Autodesk Inventor part; units mm, degrees
(part 2 of 2)
  circle A1101 centre (-5.5, 0.5) radius 0.125
  circle A1102 centre (-5.5, 1) radius 0.125
  circle A1103 centre (-5.5, 1.5) radius 0.125
  circle A1104 centre (-5.5, 2) radius 0.125
  circle A1105 centre (-5.5, 2.5) radius 0.125
  circle A1106 centre (-5.5, 3) radius 0.125
  circle A1107 centre (-5.5, 5) radius 0.125
  circle A1108 centre (-5.5, 5.5) radius 0.125
  circle A1109 centre (-5.5, 6) radius 0.125
  circle A1110 centre (-5.5, 6.5) radius 0.125
  line L13 (-6, -9) -> (-6, 0) construction
  circle A1111 centre (-6, -5.5) radius 0.125
  circle A1112 centre (-6, -5) radius 0.125
  circle A1113 centre (-6, -3.5) radius 0.125
  circle A1114 centre (-6, -4) radius 0.125
  circle A1115 centre (-6, -4.5) radius 0.125
  circle A1116 centre (-6, -7.5) radius 0.125
  circle A1117 centre (-6, -7) radius 0.125
  circle A1118 centre (-6, -6.5) radius 0.125
  circle A1119 centre (-6, -6) radius 0.125
  circle A1120 centre (-6, -3) radius 0.125
  circle A1121 centre (-6, -2.5) radius 0.125
  circle A1122 centre (-6, -2) radius 0.125
  circle A1123 centre (-6, -1.5) radius 0.125
  circle A1124 centre (-6, 0) radius 0.125
  circle A1125 centre (-6, -0.5) radius 0.125
  circle A1126 centre (-6, -1) radius 0.125
  circle A1127 centre (-6, -9) radius 0.125
  circle A1128 centre (-6, -8.5) radius 0.125
  circle A1129 centre (-6, -8) radius 0.125
  circle A1130 centre (-6, 3.5) radius 0.125
  circle A1131 centre (-6, 4) radius 0.125
  circle A1132 centre (-6, 4.5) radius 0.125
  circle A1133 centre (-6, 7) radius 0.125
  circle A1134 centre (-6, 7.5) radius 0.125
  circle A1135 centre (-6, 8) radius 0.125
  circle A1136 centre (-6, 8.5) radius 0.125
  circle A1137 centre (-6, 9) radius 0.125
  circle A1138 centre (-6, 0.5) radius 0.125
  circle A1139 centre (-6, 1) radius 0.125
  circle A1140 centre (-6, 1.5) radius 0.125
  circle A1141 centre (-6, 2) radius 0.125
  circle A1142 centre (-6, 2.5) radius 0.125
  circle A1143 centre (-6, 3) radius 0.125
  circle A1144 centre (-6, 5) radius 0.125
  circle A1145 centre (-6, 5.5) radius 0.125
  circle A1146 centre (-6, 6) radius 0.125
  circle A1147 centre (-6, 6.5) radius 0.125
  line L14 (-6.5, -9) -> (-6.5, 0) construction
  circle A1148 centre (-6.5, -5.5) radius 0.125
  circle A1149 centre (-6.5, -5) radius 0.125
  circle A1150 centre (-6.5, -3.5) radius 0.125
  circle A1151 centre (-6.5, -4) radius 0.125
  circle A1152 centre (-6.5, -4.5) radius 0.125
  circle A1153 centre (-6.5, -7.5) radius 0.125
  circle A1154 centre (-6.5, -7) radius 0.125
  circle A1155 centre (-6.5, -6.5) radius 0.125
  circle A1156 centre (-6.5, -6) radius 0.125
  circle A1157 centre (-6.5, -3) radius 0.125
  circle A1158 centre (-6.5, -2.5) radius 0.125
  circle A1159 centre (-6.5, -2) radius 0.125
  circle A1160 centre (-6.5, -1.5) radius 0.125
  circle A1161 centre (-6.5, 0) radius 0.125
  circle A1162 centre (-6.5, -0.5) radius 0.125
  circle A1163 centre (-6.5, -1) radius 0.125
  circle A1164 centre (-6.5, -9) radius 0.125
  circle A1165 centre (-6.5, -8.5) radius 0.125
  circle A1166 centre (-6.5, -8) radius 0.125
  circle A1167 centre (-6.5, 3.5) radius 0.125
  circle A1168 centre (-6.5, 4) radius 0.125
  circle A1169 centre (-6.5, 4.5) radius 0.125
  circle A1170 centre (-6.5, 7) radius 0.125
  circle A1171 centre (-6.5, 7.5) radius 0.125
  circle A1172 centre (-6.5, 8) radius 0.125
  circle A1173 centre (-6.5, 8.5) radius 0.125
  circle A1174 centre (-6.5, 9) radius 0.125
  circle A1175 centre (-6.5, 0.5) radius 0.125
  circle A1176 centre (-6.5, 1) radius 0.125
  circle A1177 centre (-6.5, 1.5) radius 0.125
  circle A1178 centre (-6.5, 2) radius 0.125
  circle A1179 centre (-6.5, 2.5) radius 0.125
  circle A1180 centre (-6.5, 3) radius 0.125
  circle A1181 centre (-6.5, 5) radius 0.125
  circle A1182 centre (-6.5, 5.5) radius 0.125
  circle A1183 centre (-6.5, 6) radius 0.125
  circle A1184 centre (-6.5, 6.5) radius 0.125
  line L15 (-7, -9) -> (-7, 0) construction
  circle A1185 centre (-7, -5.5) radius 0.125
  circle A1186 centre (-7, -5) radius 0.125
  circle A1187 centre (-7, -3.5) radius 0.125
  circle A1188 centre (-7, -4) radius 0.125
  circle A1189 centre (-7, -4.5) radius 0.125
  circle A1190 centre (-7, -7.5) radius 0.125
  circle A1191 centre (-7, -7) radius 0.125
  circle A1192 centre (-7, -6.5) radius 0.125
  circle A1193 centre (-7, -6) radius 0.125
  circle A1194 centre (-7, -3) radius 0.125
  circle A1195 centre (-7, -2.5) radius 0.125
  circle A1196 centre (-7, -2) radius 0.125
  circle A1197 centre (-7, -1.5) radius 0.125
  circle A1198 centre (-7, 0) radius 0.125
  circle A1199 centre (-7, -0.5) radius 0.125
  circle A1200 centre (-7, -1) radius 0.125
  circle A1201 centre (-7, -9) radius 0.125
  circle A1202 centre (-7, -8.5) radius 0.125
  circle A1203 centre (-7, -8) radius 0.125
  circle A1204 centre (-7, 3.5) radius 0.125
  circle A1205 centre (-7, 4) radius 0.125
  circle A1206 centre (-7, 4.5) radius 0.125
  circle A1207 centre (-7, 7) radius 0.125
  circle A1208 centre (-7, 7.5) radius 0.125
  circle A1209 centre (-7, 8) radius 0.125
  circle A1210 centre (-7, 8.5) radius 0.125
  circle A1211 centre (-7, 9) radius 0.125
  circle A1212 centre (-7, 0.5) radius 0.125
  circle A1213 centre (-7, 1) radius 0.125
  circle A1214 centre (-7, 1.5) radius 0.125
  circle A1215 centre (-7, 2) radius 0.125
  circle A1216 centre (-7, 2.5) radius 0.125
  circle A1217 centre (-7, 3) radius 0.125
  circle A1218 centre (-7, 5) radius 0.125
  circle A1219 centre (-7, 5.5) radius 0.125
  circle A1220 centre (-7, 6) radius 0.125
  circle A1221 centre (-7, 6.5) radius 0.125
  line L16 (-7.5, -9) -> (-7.5, 0) construction
  circle A1222 centre (-7.5, -5.5) radius 0.125
  circle A1223 centre (-7.5, -5) radius 0.125
  circle A1224 centre (-7.5, -3.5) radius 0.125
  circle A1225 centre (-7.5, -4) radius 0.125
  circle A1226 centre (-7.5, -4.5) radius 0.125
  circle A1227 centre (-7.5, -7.5) radius 0.125
  circle A1228 centre (-7.5, -7) radius 0.125
  circle A1229 centre (-7.5, -6.5) radius 0.125
  circle A1230 centre (-7.5, -6) radius 0.125
  circle A1231 centre (-7.5, -3) radius 0.125
  circle A1232 centre (-7.5, -2.5) radius 0.125
  circle A1233 centre (-7.5, -2) radius 0.125
  circle A1234 centre (-7.5, -1.5) radius 0.125
  circle A1235 centre (-7.5, 0) radius 0.125
  circle A1236 centre (-7.5, -0.5) radius 0.125
  circle A1237 centre (-7.5, -1) radius 0.125
  circle A1238 centre (-7.5, -9) radius 0.125
  circle A1239 centre (-7.5, -8.5) radius 0.125
  circle A1240 centre (-7.5, -8) radius 0.125
  circle A1241 centre (-7.5, 3.5) radius 0.125
  circle A1242 centre (-7.5, 4) radius 0.125
  circle A1243 centre (-7.5, 4.5) radius 0.125
  circle A1244 centre (-7.5, 7) radius 0.125
  circle A1245 centre (-7.5, 7.5) radius 0.125
  circle A1246 centre (-7.5, 8) radius 0.125
  circle A1247 centre (-7.5, 8.5) radius 0.125
  circle A1248 centre (-7.5, 9) radius 0.125
  circle A1249 centre (-7.5, 0.5) radius 0.125
  circle A1250 centre (-7.5, 1) radius 0.125
  circle A1251 centre (-7.5, 1.5) radius 0.125
  circle A1252 centre (-7.5, 2) radius 0.125
  circle A1253 centre (-7.5, 2.5) radius 0.125
  circle A1254 centre (-7.5, 3) radius 0.125
  circle A1255 centre (-7.5, 5) radius 0.125
  circle A1256 centre (-7.5, 5.5) radius 0.125
  circle A1257 centre (-7.5, 6) radius 0.125
  circle A1258 centre (-7.5, 6.5) radius 0.125
  line L17 (-8, -9) -> (-8, 0) construction
  circle A1259 centre (-8, -5.5) radius 0.125
  circle A1260 centre (-8, -5) radius 0.125
  circle A1261 centre (-8, -3.5) radius 0.125
  circle A1262 centre (-8, -4) radius 0.125
  circle A1263 centre (-8, -4.5) radius 0.125
  circle A1264 centre (-8, -7.5) radius 0.125
  circle A1265 centre (-8, -7) radius 0.125
  circle A1266 centre (-8, -6.5) radius 0.125
  circle A1267 centre (-8, -6) radius 0.125
  circle A1268 centre (-8, -3) radius 0.125
  circle A1269 centre (-8, -2.5) radius 0.125
  circle A1270 centre (-8, -2) radius 0.125
  circle A1271 centre (-8, -1.5) radius 0.125
  circle A1272 centre (-8, 0) radius 0.125
  circle A1273 centre (-8, -0.5) radius 0.125
  circle A1274 centre (-8, -1) radius 0.125
  circle A1275 centre (-8, -9) radius 0.125
  circle A1276 centre (-8, -8.5) radius 0.125
  circle A1277 centre (-8, -8) radius 0.125
  circle A1278 centre (-8, 3.5) radius 0.125
  circle A1279 centre (-8, 4) radius 0.125
  circle A1280 centre (-8, 4.5) radius 0.125
  circle A1281 centre (-8, 7) radius 0.125
  circle A1282 centre (-8, 7.5) radius 0.125
  circle A1283 centre (-8, 8) radius 0.125
  circle A1284 centre (-8, 8.5) radius 0.125
  circle A1285 centre (-8, 9) radius 0.125
  circle A1286 centre (-8, 0.5) radius 0.125
  circle A1287 centre (-8, 1) radius 0.125
  circle A1288 centre (-8, 1.5) radius 0.125
  circle A1289 centre (-8, 2) radius 0.125
  circle A1290 centre (-8, 2.5) radius 0.125
  circle A1291 centre (-8, 3) radius 0.125
  circle A1292 centre (-8, 5) radius 0.125
  circle A1293 centre (-8, 5.5) radius 0.125
  circle A1294 centre (-8, 6) radius 0.125
  circle A1295 centre (-8, 6.5) radius 0.125
  line L18 (-8.5, -9) -> (-8.5, 0) construction
  circle A1296 centre (-8.5, -5.5) radius 0.125
  circle A1297 centre (-8.5, -5) radius 0.125
  circle A1298 centre (-8.5, -3.5) radius 0.125
  circle A1299 centre (-8.5, -4) radius 0.125
  circle A1300 centre (-8.5, -4.5) radius 0.125
  circle A1301 centre (-8.5, -7.5) radius 0.125
  circle A1302 centre (-8.5, -7) radius 0.125
  circle A1303 centre (-8.5, -6.5) radius 0.125
  circle A1304 centre (-8.5, -6) radius 0.125
  circle A1305 centre (-8.5, -3) radius 0.125
  circle A1306 centre (-8.5, -2.5) radius 0.125
  circle A1307 centre (-8.5, -2) radius 0.125
  circle A1308 centre (-8.5, -1.5) radius 0.125
  circle A1309 centre (-8.5, 0) radius 0.125
  circle A1310 centre (-8.5, -0.5) radius 0.125
  circle A1311 centre (-8.5, -1) radius 0.125
  circle A1312 centre (-8.5, -9) radius 0.125
  circle A1313 centre (-8.5, -8.5) radius 0.125
  circle A1314 centre (-8.5, -8) radius 0.125
  circle A1315 centre (-8.5, 3.5) radius 0.125
  circle A1316 centre (-8.5, 4) radius 0.125
  circle A1317 centre (-8.5, 4.5) radius 0.125
  circle A1318 centre (-8.5, 7) radius 0.125
  circle A1319 centre (-8.5, 7.5) radius 0.125
  circle A1320 centre (-8.5, 8) radius 0.125
  circle A1321 centre (-8.5, 8.5) radius 0.125
  circle A1322 centre (-8.5, 9) radius 0.125
  circle A1323 centre (-8.5, 0.5) radius 0.125
  circle A1324 centre (-8.5, 1) radius 0.125
  circle A1325 centre (-8.5, 1.5) radius 0.125
  circle A1326 centre (-8.5, 2) radius 0.125
  circle A1327 centre (-8.5, 2.5) radius 0.125
  circle A1328 centre (-8.5, 3) radius 0.125
  circle A1329 centre (-8.5, 5) radius 0.125
  circle A1330 centre (-8.5, 5.5) radius 0.125
  circle A1331 centre (-8.5, 6) radius 0.125
  circle A1332 centre (-8.5, 6.5) radius 0.125
  line L19 (-9, -9) -> (-9, 0) construction
  circle A1333 centre (-9, -5.5) radius 0.125
  circle A1334 centre (-9, -5) radius 0.125
  circle A1335 centre (-9, -3.5) radius 0.125
  circle A1336 centre (-9, -4) radius 0.125
  circle A1337 centre (-9, -4.5) radius 0.125
  circle A1338 centre (-9, -7.5) radius 0.125
  circle A1339 centre (-9, -7) radius 0.125
  circle A1340 centre (-9, -6.5) radius 0.125
  circle A1341 centre (-9, -6) radius 0.125
  circle A1342 centre (-9, -3) radius 0.125
  circle A1343 centre (-9, -2.5) radius 0.125
  circle A1344 centre (-9, -2) radius 0.125
  circle A1345 centre (-9, -1.5) radius 0.125
  circle A1346 centre (-9, 0) radius 0.125
  circle A1347 centre (-9, -0.5) radius 0.125
  circle A1348 centre (-9, -1) radius 0.125
  circle A1349 centre (-9, -9) radius 0.125
  circle A1350 centre (-9, -8.5) radius 0.125
  circle A1351 centre (-9, -8) radius 0.125
  circle A1352 centre (-9, 3.5) radius 0.125
  circle A1353 centre (-9, 4) radius 0.125
  circle A1354 centre (-9, 4.5) radius 0.125
  circle A1355 centre (-9, 7) radius 0.125
  circle A1356 centre (-9, 7.5) radius 0.125
  circle A1357 centre (-9, 8) radius 0.125
  circle A1358 centre (-9, 8.5) radius 0.125
  circle A1359 centre (-9, 9) radius 0.125
  circle A1360 centre (-9, 0.5) radius 0.125
  circle A1361 centre (-9, 1) radius 0.125
  circle A1362 centre (-9, 1.5) radius 0.125
  circle A1363 centre (-9, 2) radius 0.125
  circle A1364 centre (-9, 2.5) radius 0.125
  circle A1365 centre (-9, 3) radius 0.125
  circle A1366 centre (-9, 5) radius 0.125
  circle A1367 centre (-9, 5.5) radius 0.125
  circle A1368 centre (-9, 6) radius 0.125
  circle A1369 centre (-9, 6.5) radius 0.125
  dimension "d8" = 0.25
  constraints: 1369 centre point, 40 end point, 2 point on circle, 1 perpendicular, 1 vertical alignment
  measures "d8" diameter of A0
